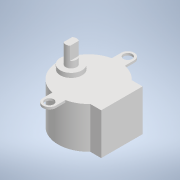
# Autodesk Inventor part: smol stepper
Saved by Autodesk Inventor 2022 (Build 260153000, 153)
## iProperties
Created: 2021-12-07
Part Number: smol stepper
Material: Generic
Document SubType Name: Modeling
Designer: efred
Density: 1 g/cm^3
Appearance: Default
Author: efred
Autodesk Inventor part; units mm, degrees
ref_plane "YZ Plane" through (0, 0, 0) normal (1, 0, 0) x (0, 1, 0)
ref_plane "XZ Plane" through (0, 0, 0) normal (0, 1, 0) x (-1, 0, 0)
ref_plane "XY Plane" through (0, 0, 0) normal (0, 0, 1) x (1, 0, 0)
sketch "Sketch1" plane through (0, 0, 0) normal (0, 1, 0) x (-1, 0, 0)
  circle A0 centre (0, 0) radius 14
  line L0 (-10.2835, 9.5) -> (-15.2835, 9.5)
  line L1 (-15.2835, 9.5) -> (-15.2835, -9.5)
  line L2 (-15.2835, -9.5) -> (-10.2835, -9.5)
  line L3 (-10.2835, -9.5) -> (-10.2835, 9.5)
  point P0 (-10.2835, 0)
  dimension "d0" = 28
  dimension "d3" = 5
  dimension "d4" = 19
  constraints: 8 end point, 2 parallel, 2 point on circle, 1 centre point, 1 coincident, 1 horizontal, 1 horizontal alignment, 1 midpoint, 1 perpendicular
  measures "d0" diameter of A0
  measures "d3" distance of L0.start L0.end
  measures "d4" distance between parallel lines of L0 L2
extrude "Extrusion1" add sketch "Sketch1" along normal mid plane 19
sketch "Sketch2" plane through (0, 9.5, 0) normal (0, 1, 0) x (1, 0, 0)
  line L0 (0, 0) -> (15.2835, 0) construction
  line L1 (15.2835, -9.5) -> (15.2835, 9.5) projected
  circle A0 centre (0, 18) radius 2
  arc A1 (10.2835, 9.5) -> (10.2835, -9.5) centre (0, 0) ccw projected
  line L2 (-3, 13.6748) -> (3, 13.6748)
  line L3 (3, 13.6748) -> (3, 18)
  line L4 (3, 18) -> (-3, 18) construction
  line L5 (-3, 18) -> (-3, 13.6748)
  arc A2 (3, 18) -> (-3, 18) centre (0, 18) ccw
  circle A3 centre (0, -18) radius 2
  line L6 (-3, -13.6748) -> (3, -13.6748)
  line L7 (3, -13.6748) -> (3, -18)
  line L8 (3, -18) -> (-3, -18) construction
  line L9 (-3, -18) -> (-3, -13.6748)
  arc A4 (-3, -18) -> (3, -18) centre (0, -18) ccw
  point P0 (0, 14)
  point P1 (0, 13.6748)
  point P2 (0, -14)
  point P3 (0, -13.6748)
  dimension "d5" = 4
  dimension "d6" = 4
  dimension "d7" = 3
  constraints: 18 end point, 8 symmetric about line, 7 point on circle, 4 centre point, 3 vertical alignment, 2 midpoint, 2 parallel, 2 tangent, 1 concentric, 1 horizontal, 1 perpendicular, 2 other
  measures "d5" diameter of A0
  measures "d6" distance of point (0, 14) A0.centre
  measures "d7" distance of A0.centre L4.end
extrude "Extrusion2" add sketch "Sketch2" against normal blind 1 contours A1 L7 A4 L9 | A1 L5 A2 L3
sketch "Sketch3" plane through (0, 9.5, 0) normal (0, 1, 0) x (1, 0, 0)
  circle A0 centre (-8, 0) radius 5
  arc A1 (-3, 13.6748) -> (-3, -13.6748) centre (0, 0) ccw projected
  point P0 (-14, 0)
  point P1 (-14, 0)
  dimension "d10" = 10
  dimension "d11" = 6
  constraints: 3 horizontal alignment, 2 point on circle, 1 centre point
  measures "d10" diameter of A0
  measures "d11" distance of point (-14, 0) A0.centre
extrude "Extrusion3" add sketch "Sketch3" along normal blind 2
sketch "Sketch4" plane through (-8, 11.5, 0) normal (0, 1, 0) x (1, 0, 0)
  circle A0 centre (0, 0) radius 2.5
  circle A1 centre (0, 0) radius 5 projected
  point P0 (8, 0)
  dimension "d14" = 5
  constraints: 1 centre point, 1 concentric
  measures "d14" diameter of A0
extrude "Extrusion4" add sketch "Sketch4" along normal blind 9 contours A0
sketch "Sketch5" plane through (-8, 20.5, 0) normal (0, 1, 0) x (1, 0, 0)
  circle A0 centre (0, 0) radius 2.5 projected
  circle A1 centre (0, 0) radius 2.5 projected
  line L0 (1.5, -2) -> (1.5, 2)
  line L1 (0, -2.5) -> (0, 2.5) construction
  line L2 (-1.5, -2) -> (-1.5, 2)
  point P0 (8, 0)
  dimension "d19" = 3
  constraints: 6 end point, 4 point on circle, 2 symmetric about line, 1 midpoint, 1 parallel, 1 vertical
  measures "d19" distance between parallel lines of L0 L2
extrude "Extrusion5" cut sketch "Sketch5" against normal blind 6 contours A0 L0 | L2 A0
body "Solid1"
